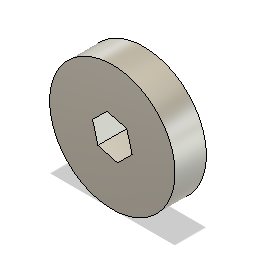
Shooter+Side (Autodesk Fusion 360 archive; units mm, degrees)
design "Shooter Wheel"
Autodesk Fusion 360 part; units mm, degrees
sketch "Sketch1" plane through (0, 0, 0) normal (0, 0, 1) x (1, 0, 0)
  circle A0 centre (0, 0) radius 25.4
  line L0 (8.0129, -2.1471) -> (5.8659, 5.8659)
  line L1 (5.8659, 5.8659) -> (-2.1471, 8.0129)
  line L2 (-2.1471, 8.0129) -> (-8.0129, 2.1471)
  line L3 (-8.0129, 2.1471) -> (-5.8659, -5.8659)
  line L4 (-5.8659, -5.8659) -> (2.1471, -8.0129)
  line L5 (2.1471, -8.0129) -> (8.0129, -2.1471)
  dimension "d1" = 50.8
  constraint coincident A0.centre origin
  measures "d1" diameter of A0
extrude "Extrude1" add sketch "Sketch1" along normal blind 12.7
